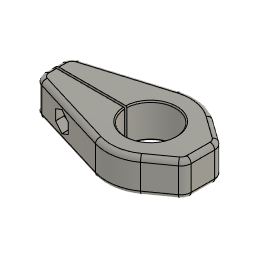
Knob_v8 (Autodesk Fusion 360 design; units mm, degrees)
Autodesk Fusion 360 part; units mm, degrees
note: some values were not read from the file. Set by a fixed rule: which sketch regions a step uses.
sketch "Sketch1" plane through (0, 0, 0) normal (0, 0, 1) x (1, 0, 0)
  circle A0 centre (0, 0) radius 11
  circle A1 centre (0, 0) radius 19.5
  line L0 (-43, 7.25) -> (-43, -7.25)
  line L1 (23, 7.5) -> (23, -7.5)
  line L2 (-43, 7.25) -> (-5.6988, 18.6487)
  line L3 (-43, -7.25) -> (-5.6988, -18.6487)
  line L4 (23, 7.5) -> (11.3657, 15.8452)
  line L5 (23, -7.5) -> (11.3657, -15.8452)
  line L6 (-31, 0) -> (-23, 0) construction
  line L7 (-19.5, 0) -> (-43, 0) construction
  line L8 (-31, 10.917) -> (-31, -10.917)
  line L9 (-10.9886, 0.5) -> (-43, 0.5)
  line L10 (-10.9886, -0.5) -> (-43, -0.5)
  line L11 (-10.9886, 0.5) -> (-10.9886, -0.5) construction
  line L12 (-11, 0) -> (-43, 0) construction
  line L13 (-31, -10.917) -> (-1.3486, -10.917) construction
  line L14 (-31, 10.917) -> (-1.3486, 10.917) construction
  point P0 (11, 0)
  point P1 (-43, 0)
  point P2 (23, 0)
  point P3 (-11, 0)
  point P4 (-19.5, 0)
  point P5 (-10.9886, 0)
  point P6 (-27, 0)
  point P7 (-27, 0)
  dimension "d1" = 22
  dimension "d2" = 8.5
  dimension "d7" = 14.5
  dimension "d8" = 15
  dimension "d9" = 12
  dimension "d14" = 8
  dimension "d15" = 12
  dimension "d16" = 3.5
  dimension "d17" = 32
  dimension "d47" = 1
  dimension "d48" = 20.0114
  constraint coincident A0.centre A1.centre
  constraint coincident A0 P0
  constraint horizontal A0.centre P0
  constraint vertical L0
  constraint midpoint L0 P1
  constraint horizontal A0.centre P1
  constraint vertical L1
  constraint midpoint L1 P2
  constraint horizontal A0.centre P2
  constraint coincident A1 L2.end
  constraint coincident A1 L3.end
  constraint tangent A1 L2
  constraint tangent A1 L3
  constraint coincident A0 P3
  constraint horizontal A0.centre P3
  constraint coincident A1 L4.end
  constraint coincident A1 L5.end
  constraint tangent A1 L5
  constraint tangent A1 L4
  constraint horizontal L6
  constraint coincident A1 P4
  constraint horizontal P3 P4
  constraint coincident P4 L7.start
  constraint coincident P1 L7.end
  constraint coincident L2 L8.start
  constraint coincident L3 L8.end
  constraint perpendicular L7 L8
  constraint coincident L6.start L8
  constraint coincident A0 L9.start
  constraint coincident L0 L9.end
  constraint perpendicular L0 L9
  constraint coincident A0 L10.start
  constraint coincident L0 L10.end
  constraint perpendicular L0 L10
  constraint midpoint L11 P5
  constraint horizontal P3 P5
  constraint coincident P3 L12.start
  constraint midpoint L12 P7
  constraint midpoint L6 P7
  constraint coincident P7 P6
  constraint coincident A0 L13.end
  constraint perpendicular L8 L13
  constraint coincident A0 L14.end
  constraint perpendicular L8 L14
  measures "d1" diameter of A0
  measures "d7" distance of L0.start L0.end
  measures "d8" distance of L1.start L1.end
  measures "d9" distance of P0 P2
  measures "d14" distance of L6.start L6.end
  measures "d15" distance of P1 L6.start
  measures "d16" distance of L6.end P4
  measures "d17" distance of L0 P3
  measures "d47" distance of L9 L10
  measures "d48" distance of L8 P5
extrude "Extrude1" add sketch "Sketch1" along normal blind 15 contours A0 A1 L9 L10 | A1 L2 L8 L9 | A1 L3 L8 L10 | L0 L2 L8 L9 | L0 L3 L8 L10 | A1 L1 L4 L5 picked at (-9.972, 13.3152)
sketch "Sketch2" plane through (0, 0, 0) normal (0, 1, 0) x (1, 0, 0)
  line L0 (-19.5, 0) -> (-43, 0)
  line L1 (-43, -15) -> (-5.6988, -15) construction
  circle A0 centre (-27, -7.5) radius 2.4
  line L2 (-23, -5.1906) -> (-27, -2.8812)
  line L3 (-27, -2.8812) -> (-31, -5.1906)
  line L4 (-31, -5.1906) -> (-31, -9.8094)
  line L5 (-31, -9.8094) -> (-27, -12.1188)
  line L6 (-27, -12.1188) -> (-23, -9.8094)
  line L7 (-23, -9.8094) -> (-23, -5.1906)
  line L8 (-43, 0) -> (-5.6988, 0) construction
  line L9 (-5.6988, 0) -> (-5.6988, -15) construction
  line L10 (-5.6988, -15) -> (-43, -15) construction
  line L11 (-43, -15) -> (-43, 0) construction
  line L12 (-31, -15) -> (-31, 0) construction
  line L13 (-43, 0) -> (-5.6988, 0) construction
  circle A1 centre (-27, -7.5) radius 4.15
  line L14 (-27, 0) -> (-27, -15) construction
  point P0 (-31.25, 0)
  point P1 (-27, -7.5)
  point P2 (-27, -7.5)
  point P3 (-31, 0)
  point P4 (-27, 0)
  point P5 (-27, -7.5)
  dimension "d24" = 4.8
  dimension "d25" = 4
  dimension "d39" = 8.3
  constraint midpoint L0 P0
  constraint coincident P5 P2
  constraint vertical L7
  constraint coincident L1 L12.start
  constraint perpendicular L0 L12
  constraint coincident P3 L13
  constraint collinear L4 L12
  constraint concentric A0 A1
  constraint coincident P4 L14.start
  constraint coincident L1 L14.end
  constraint perpendicular L1 L14
  constraint midpoint L14 P5
  measures "d24" diameter of A0
  measures "d25" distance of P5 L7
  measures "d39" diameter of A1
ref_plane "WorkPlane3" through (-16.1743, -10.917, 0) normal (0, -1, 0) x (1, 0, 0)
ref_plane "WorkPlane4" through (-16.1743, 10.917, 0) normal (0, -1, 0) x (1, 0, 0)
extrude "Extrude3" cut sketch "Sketch2" along normal blind 3.75 and the other way blind 30 from surface at -10.917 contours A0 | L2 L7 A1 | L2 L3 L4 L5 L6 L7 A1 | L2 L3 A1 | L6 L7 A1 | L3 L4 A1 | L5 L6 A1 | L4 L5 A1
extrude "Extrude4" cut sketch "Sketch2" along normal mid plane 40 contours A0
extrude "Extrude5" cut sketch "Sketch2" along normal blind 8.5 and the other way blind 4 from surface at 10.917 contours A0 | L2 L3 L4 L5 L6 L7 A1 | L2 A1 | L7 A1 | L3 A1 | L6 A1 | L4 A1 | L5 A1
sketch "Sketch3" plane through (0, 0, 15) normal (0, 0, 1) x (-1, 0, 0)
  arc A0 (10.9886, 0.5) -> (10.9886, -0.5) centre (0, 0) ccw
  line L0 (10.9886, 0.5) -> (43, 0.5)
  line L1 (43, 0.5) -> (43, 7.25)
  line L2 (43, 7.25) -> (5.6988, 18.6487)
  arc A1 (5.6988, 18.6487) -> (-11.3657, 15.8452) centre (0, 0) ccw
  line L3 (-11.3657, 15.8452) -> (-23, 7.5)
  line L4 (-23, 7.5) -> (-23, -7.5)
  line L5 (-23, -7.5) -> (-11.3657, -15.8452)
  arc A2 (-11.3657, -15.8452) -> (5.6988, -18.6487) centre (0, 0) ccw
  line L6 (5.6988, -18.6487) -> (43, -7.25)
  line L7 (43, -7.25) -> (43, -0.5)
  line L8 (43, -0.5) -> (10.9886, -0.5)
fillet "Fillet1" radius 4.5 4 edges at (-43, -7.25, 7.5) (23, -7.5, 7.5) (23, 7.5, 7.5) (-43, 7.25, 7.5)
fillet "Fillet2" radius 2 26 edges at (16.2443, -12.3458, 15) (22.5033, -7.245, 15) (23, 0, 15) (22.5033, 7.245, 15) (16.2443, 12.3458, 15) (3.1612, 19.2421, 15) (-22.7569, 13.436, 15) (-42.1172, 6.5967, 15) (-43, 2.2099, 15) (-43, -2.2099, 15) (-42.1172, -6.5967, 15) (-22.7569, -13.436, 15) (3.1612, -19.2421, 15) (16.2443, -12.3458, 0) (22.5033, -7.245, 0) (23, 0, 0) (22.5033, 7.245, 0) (16.2443, 12.3458, 0) (3.1612, 19.2421, 0) (-22.7569, 13.436, 0) (-42.1172, 6.5967, 0) (-43, 2.2099, 0) (-43, -2.2099, 0) (-42.1172, -6.5967, 0) (-22.7569, -13.436, 0) (3.1612, -19.2421, 0)
fillet "Fillet3" radius 0.5 2 edges at (11, 0, 15) (11, 0, 0)
sketch "Sketch6" plane through (0, 0, 15) normal (0, 0, 1) x (-1, 0, 0)
  line L0 (43, 0.5) -> (43, 7.25)
  line L1 (43, 7.25) -> (5.6988, 18.6487)
  arc A0 (5.6988, 18.6487) -> (-11.3657, 15.8452) centre (0, 0) ccw
  line L2 (-11.3657, 15.8452) -> (-23, 7.5)
  line L3 (-23, 7.5) -> (-23, -7.5)
  line L4 (-23, -7.5) -> (-11.3657, -15.8452)
  arc A1 (-11.3657, -15.8452) -> (5.6988, -18.6487) centre (0, 0) ccw
  line L5 (5.6988, -18.6487) -> (43, -7.25)
  line L6 (43, -7.25) -> (43, -0.5)
  line L7 (43, 0.5) -> (43, -0.5)
  line L8 (-23, 1.25) -> (-23.5, 0)
  line L9 (-23.5, 0) -> (-23, -1.25)
  line L10 (-23, 1.25) -> (-23, -1.25)
  point P0 (-23, 0)
  dimension "d60" = 0.5
  dimension "d61" = 2.5
  constraint coincident L0.start L7.start
  constraint coincident L6.end L7.end
  constraint coincident L3 L8.start
  constraint coincident L3 L9.end
  constraint midpoint L10 P0
  constraint horizontal A0.centre P0
  constraint equal L8 L9
  measures "d60" distance of L8.end P0
  measures "d61" distance of L8.start L9.end
equation "d25 = ( 8 / 2 ) * 1 mm"
